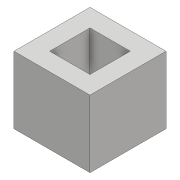
# Autodesk Inventor part: Part1
Saved by Autodesk Inventor 2017 (Build 210142000, 142)
## iProperties
Created: 2019-07-22
Part Number: Part1
Material: Generic
Document SubType Name: Modeling
Designer: Admin
Density: 1 g/cm^3
Appearance: Default
Author: Admin
Autodesk Inventor part; units mm, degrees
ref_plane "YZ Plane" through (0, 0, 0) normal (1, 0, 0) x (0, 1, 0)
ref_plane "XZ Plane" through (0, 0, 0) normal (0, 1, 0) x (-1, 0, 0)
ref_plane "XY Plane" through (0, 0, 0) normal (0, 0, 1) x (1, 0, 0)
ref_plane "Work Plane1" through (0, 0, 20) normal (0, 0, 1) x (1, 0, 0)
sketch "Sketch2" plane through (0, 0, 20) normal (0, 0, 1) x (1, 0, 0)
  line L0 (4.5, -4.5) -> (-4.5, -4.5)
  line L1 (-4.5, -4.5) -> (-4.5, 4.5)
  line L2 (-4.5, 4.5) -> (4.5, 4.5)
  line L3 (4.5, 4.5) -> (4.5, -4.5)
  line L4 (4.5, -4.5) -> (-4.5, 4.5) construction
  line L5 (-4.5, -4.5) -> (4.5, 4.5) construction
  line L6 (8.4853, -8.4853) -> (-8.4853, -8.4853)
  line L7 (-8.4853, -8.4853) -> (-8.4853, 8.4853)
  line L8 (-8.4853, 8.4853) -> (8.4853, 8.4853)
  line L9 (8.4853, 8.4853) -> (8.4853, -8.4853)
  line L10 (8.4853, -8.4853) -> (-8.4853, 8.4853) construction
  line L11 (-8.4853, -8.4853) -> (8.4853, 8.4853) construction
  point P0 (0, 0)
  dimension "d4" = 9
  dimension "d5" = 9
  constraints: 24 end point, 4 midpoint, 4 parallel, 2 horizontal, 2 perpendicular
  measures "d4" distance of L1.end L2.end
  measures "d5" distance of L0.end L1.end
extrude "Extrusion2" add sketch "Sketch2" along normal blind 10 and the other way blind 5
body "Solid1"
body "Solid2"
